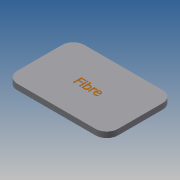
# Autodesk Inventor part: pullbox
Saved by Autodesk Inventor 2016 (Build 200138000, 138)
## iProperties
Created: 2014-12-12
Part Number: pullbox
Material: ABS Plastic
Document SubType Name: Modeling
Designer: Dave
Density: 1.06 g/cm^3
Appearance: Smooth - White
Author: Dave
Autodesk Inventor part; units mm, degrees
ref_plane "YZ Plane" through (0, 0, 0) normal (1, 0, 0) x (0, 1, 0)
ref_plane "XZ Plane" through (0, 0, 0) normal (0, 1, 0) x (-1, 0, 0)
ref_plane "XY Plane" through (0, 0, 0) normal (0, 0, 1) x (1, 0, 0)
sketch "Sketch1" plane through (0, 0, 0) normal (0, 1, 0) x (-1, 0, 0)
  line L0 (101.6, 0) -> (812.8, 0)
  line L1 (914.4, 101.6) -> (914.4, 508)
  line L2 (812.8, 609.6) -> (101.6, 609.6)
  line L3 (0, 508) -> (0, 101.6)
  arc A0 (101.6, 609.6) -> (0, 508) centre (101.6, 508) ccw
  arc A1 (0, 101.6) -> (101.6, 0) centre (101.6, 101.6) ccw
  arc A2 (812.8, 0) -> (914.4, 101.6) centre (812.8, 101.6) ccw
  arc A3 (914.4, 508) -> (812.8, 609.6) centre (812.8, 508) ccw
  point P0 (0, 0)
  point P1 (914.4, 609.6)
  point P2 (914.4, 0)
  point P3 (0, 609.6)
  dimension "d0" = 914.4
  dimension "d1" = 609.6
  dimension "d9" = 101.6
  constraints: 8 end point, 8 point on circle, 8 point on line, 8 tangent, 4 centre point, 3 equal radius, 2 parallel, 1 horizontal, 1 perpendicular
  measures "d0" distance of point (0, 609.6) point (914.4, 609.6)
  measures "d1" distance of point (914.4, 609.6) point (914.4, 0)
  measures "d9" radius of A0
extrude "Extrusion1" add sketch "Sketch1" along normal blind 50.8
sketch "Sketch8" plane through (0, 50.8, 0) normal (0, 1, 0) x (1, 0, 0)
  line L0 (-577.5208, -267.3319) -> (-568.3422, -267.3319) construction
  line L1 (-568.3422, -267.3319) -> (-568.3422, -270.58) construction
  line L2 (-568.3422, -270.58) -> (-577.5208, -270.58) construction
  line L3 (-577.5208, -270.58) -> (-577.5208, -267.3319) construction
  line L4 (-524.2302, -279.7438) -> (-559.6749, -279.7438)
  line L5 (-559.6749, -279.7438) -> (-559.6749, -301.2329)
  line L6 (-559.6749, -301.2329) -> (-525.7122, -301.2329)
  line L7 (-525.7122, -301.2329) -> (-525.7122, -310.2485)
  line L8 (-525.7122, -310.2485) -> (-559.6749, -310.2485)
  line L9 (-559.6749, -310.2485) -> (-559.6749, -346.9282)
  line L10 (-559.6749, -346.9282) -> (-569.802, -346.9282)
  line L11 (-569.802, -346.9282) -> (-569.802, -270.7282)
  line L12 (-569.802, -270.7282) -> (-524.2302, -270.7282)
  line L13 (-524.2302, -270.7282) -> (-524.2302, -279.7438)
  line L14 (-506.0756, -346.9282) -> (-515.7086, -346.9282)
  line L15 (-515.7086, -346.9282) -> (-515.7086, -289.7473)
  line L16 (-515.7086, -289.7473) -> (-506.0756, -289.7473)
  line L17 (-506.0756, -289.7473) -> (-506.0756, -346.9282)
  line L18 (-505.3963, -280.2378) -> (-516.3261, -280.2378)
  line L19 (-516.3261, -280.2378) -> (-516.3261, -270.2342)
  line L20 (-516.3261, -270.2342) -> (-505.3963, -270.2342)
  line L21 (-505.3963, -270.2342) -> (-505.3963, -280.2378)
  spline S0 degree 2 poles (-444.0164, -317.4115) (-444.0164, -331.4289) (-457.6015, -348.5337) (-467.8521, -348.5337) knots 0 0 0 1 2 2 2
  spline S1 degree 2 poles (-467.8521, -348.5337) (-472.4834, -348.5337) (-479.0907, -346.249) (-482.3017, -344.2729) knots 0 0 0 1 2 2 2
  line L22 (-482.3017, -344.2729) -> (-482.9192, -346.9282)
  line L23 (-482.9192, -346.9282) -> (-491.9347, -346.9282)
  line L24 (-491.9347, -346.9282) -> (-491.9347, -267.3319)
  line L25 (-491.9347, -267.3319) -> (-482.3017, -267.3319)
  line L26 (-482.3017, -267.3319) -> (-482.3017, -295.7371)
  spline S2 degree 2 poles (-482.3017, -295.7371) (-478.6584, -292.4643) (-470.1986, -288.1418) (-464.8263, -288.1418) knots 0 0 0 1 2 2 2
  spline S3 degree 2 poles (-464.8263, -288.1418) (-455.1315, -288.1418) (-444.0164, -303.6412) (-444.0164, -317.4115) knots 0 0 0 1 2 2 2
  spline S4 degree 2 poles (-453.9582, -318.1525) (-453.9582, -307.902) (-460.195, -297.2809) (-467.1111, -297.2809) knots 0 0 0 1 2 2 2
  spline S5 degree 2 poles (-467.1111, -297.2809) (-471.0013, -297.2809) (-479.0289, -300.9859) (-482.3017, -303.8264) knots 0 0 0 1 2 2 2
  line L27 (-482.3017, -303.8264) -> (-482.3017, -336.6159)
  spline S6 degree 2 poles (-482.3017, -336.6159) (-478.6584, -338.4067) (-473.0391, -339.8887) (-469.7046, -339.8887) knots 0 0 0 1 2 2 2
  spline S7 degree 2 poles (-469.7046, -339.8887) (-462.3563, -339.8887) (-453.9582, -329.4528) (-453.9582, -318.1525) knots 0 0 0 1 2 2 2
  line L28 (-403.6934, -300.0596) -> (-404.1874, -300.0596)
  spline S8 degree 2 poles (-404.1874, -300.0596) (-405.2989, -299.7509) (-407.7072, -299.6274) (-409.3744, -299.6274) knots 0 0 0 1 2 2 2
  spline S9 degree 2 poles (-409.3744, -299.6274) (-413.2647, -299.6274) (-420.9218, -303.0237) (-424.3798, -306.3582) knots 0 0 0 1 2 2 2
  line L29 (-424.3798, -306.3582) -> (-424.3798, -346.9282)
  line L30 (-424.3798, -346.9282) -> (-434.0129, -346.9282)
  line L31 (-434.0129, -346.9282) -> (-434.0129, -289.7473)
  line L32 (-434.0129, -289.7473) -> (-424.3798, -289.7473)
  line L33 (-424.3798, -289.7473) -> (-424.3798, -298.2689)
  spline S10 degree 2 poles (-424.3798, -298.2689) (-419.131, -293.5759) (-411.2887, -289.7473) (-407.5837, -289.7473) knots 0 0 0 1 2 2 2
  spline S11 degree 2 poles (-407.5837, -289.7473) (-406.1017, -289.7473) (-404.6197, -289.8708) (-403.6934, -290.0561) knots 0 0 0 1 2 2 2
  line L34 (-403.6934, -290.0561) -> (-403.6934, -300.0596)
  spline S12 degree 2 poles (-371.3979, -348.225) (-385.1065, -348.225) (-400.1736, -332.8491) (-400.1736, -318.6465) knots 0 0 0 1 2 2 2
  spline S13 degree 2 poles (-400.1736, -318.6465) (-400.1736, -304.6909) (-385.5388, -288.1418) (-373.7445, -288.1418) knots 0 0 0 1 2 2 2
  spline S14 degree 2 poles (-373.7445, -288.1418) (-368.4339, -288.1418) (-360.2211, -291.2293) (-357.1954, -294.5021) knots 0 0 0 1 2 2 2
  spline S15 degree 2 poles (-357.1954, -294.5021) (-354.1078, -297.7749) (-350.8351, -307.2227) (-350.8351, -314.077) knots 0 0 0 1 2 2 2
  line L35 (-350.8351, -314.077) -> (-350.8351, -319.3258)
  line L36 (-350.8351, -319.3258) -> (-390.4171, -319.3258)
  spline S16 degree 2 poles (-390.4171, -319.3258) (-390.4171, -329.2676) (-380.4135, -339.8269) (-371.5214, -339.8269) knots 0 0 0 1 2 2 2
  spline S17 degree 2 poles (-371.5214, -339.8269) (-368.3722, -339.8269) (-362.2589, -338.4067) (-359.7889, -337.2951) knots 0 0 0 1 2 2 2
  spline S18 degree 2 poles (-359.7889, -337.2951) (-357.1954, -336.0601) (-353.6138, -333.8989) (-352.4406, -332.9109) knots 0 0 0 1 2 2 2
  line L37 (-352.4406, -332.9109) -> (-351.8848, -332.9109)
  line L38 (-351.8848, -332.9109) -> (-351.8848, -343.4084)
  spline S19 degree 2 poles (-351.8848, -343.4084) (-353.5521, -344.0877) (-358.6156, -346.0637) (-360.5916, -346.6195) knots 0 0 0 1 2 2 2
  spline S20 degree 2 poles (-360.5916, -346.6195) (-363.3704, -347.4222) (-367.9399, -348.225) (-371.3979, -348.225) knots 0 0 0 1 2 2 2
  spline S21 degree 2 poles (-360.2211, -311.9775) (-360.3446, -308.0872) (-361.9501, -302.4062) (-363.4939, -300.4919) knots 0 0 0 1 2 2 2
  spline S22 degree 2 poles (-363.4939, -300.4919) (-365.1612, -298.3306) (-370.4099, -296.0459) (-374.3002, -296.0459) knots 0 0 0 1 2 2 2
  spline S23 degree 2 poles (-374.3002, -296.0459) (-378.1287, -296.0459) (-383.501, -298.3306) (-385.724, -300.5537) knots 0 0 0 1 2 2 2
  spline S24 degree 2 poles (-385.724, -300.5537) (-387.8853, -302.8384) (-390.1083, -308.3342) (-390.4171, -311.9775) knots 0 0 0 1 2 2 2
  line L39 (-390.4171, -311.9775) -> (-360.2211, -311.9775)
  point P0 (0, 0)
  constraints: 2 other
emboss "Emboss1" sketch "Sketch8" operation add depth 2.54 direction (0, -1, 0)
body "Solid1"
